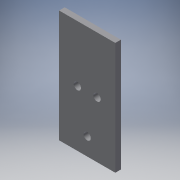
# Autodesk Inventor part: Motor cover upper
Saved by Autodesk Inventor 2019 (Build 230136000, 136)
## iProperties
Created: 2018-12-04
Part Number: Motor cover upper
Material: Generic
Document SubType Name: Modeling
Designer: Varga Daniel
Density: 1 g/cm^3
Appearance: Default
Author: Varga Daniel
Autodesk Inventor part; units mm, degrees
ref_plane "YZ Plane" through (0, 0, 0) normal (1, 0, 0) x (0, 1, 0)
ref_plane "XZ Plane" through (0, 0, 0) normal (0, 1, 0) x (-1, 0, 0)
ref_plane "XY Plane" through (0, 0, 0) normal (0, 0, 1) x (1, 0, 0)
sketch "Sketch1" plane through (0, 0, 0) normal (0, 0, 1) x (1, 0, 0)
  line L0 (13.75, 44.8) -> (-36.25, 44.8)
  line L1 (-36.25, 44.8) -> (-36.25, -55.2)
  line L2 (-36.25, -55.2) -> (13.75, -55.2)
  line L3 (13.75, -55.2) -> (13.75, 44.8)
  circle A0 centre (-2.5, -5.2) radius 2.5 construction
  circle A1 centre (-20, -5.2) radius 2.5 construction
  circle A2 centre (-11.25, -39.5) radius 2.5 construction
  circle A3 centre (-2.5, -5.2) radius 3.25
  circle A4 centre (-20, -5.2) radius 3.25
  circle A5 centre (-11.25, -39.5) radius 3.25
  point P0 (0, 0)
  dimension "d0" = 6.5
  dimension "d1" = 6.5
  dimension "d2" = 6.5
  constraints: 8 end point, 3 centre point, 3 coincident, 2 parallel, 1 horizontal, 1 perpendicular
  measures "d0" diameter of A3
  measures "d1" diameter of A4
  measures "d2" diameter of A5
extrude "Extrusion1" add sketch "Sketch1" along normal blind 3.4
body "Solid1"
